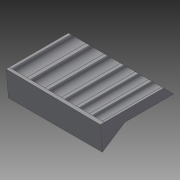
# Autodesk Inventor part: coin_holder
Saved by Autodesk Inventor 2015 (Build 190159000, 159)
## iProperties
Created: 2015-02-10
Part Number: coin_holder
Material: Generic
Document SubType Name: Modeling
Designer: Justin
Density: 1 g/cm^3
Appearance: Default
Author: Justin
Autodesk Inventor part; units mm, degrees
ref_plane "YZ Plane" through (0, 0, 0) normal (1, 0, 0) x (0, 1, 0)
ref_plane "XZ Plane" through (0, 0, 0) normal (0, 1, 0) x (-1, 0, 0)
sketch "Sketch1" plane through (0, 0, 0) normal (0, 0, 1) x (1, 0, 0)
  arc A0 (12.7973, -6.8176) -> (-12.597, -7.1809) centre (0, 0) ccw
  arc A1 (50.4829, -6.2785) -> (26.2017, -6.6259) centre (38.25, 0) ccw
  arc A2 (85.5853, -5.7763) -> (63.5844, -6.091) centre (74.5, 0) ccw
  arc A3 (117.8988, -5.314) -> (98.5072, -5.5914) centre (108.125, 0) ccw
  arc A4 (147.9764, -4.8837) -> (130.6669, -5.1313) centre (139.25, 0) ccw
  arc A5 (177.1345, -4.4665) -> (160.4967, -4.7045) centre (168.75, 0) ccw
  line L0 (-20, 20) -> (188.75, 20)
  line L1 (188.75, 20) -> (188.75, -4.3003)
  line L2 (-20, 20) -> (-20, -7.2868)
  line L3 (-20, -7.2868) -> (188.75, -4.3003)
  dimension "d0" = 29
  dimension "d1" = 27.5
  dimension "d2" = 25
  dimension "d3" = 22.25
  dimension "d4" = 20
  dimension "d5" = 19
  dimension "d6" = 38.25
  dimension "d7" = 36.25
  dimension "d8" = 33.625
  dimension "d9" = 31.125
  dimension "d10" = 29.5
  dimension "d11" = 0
  dimension "d12" = 0
  dimension "d13" = 0
  dimension "d14" = 0
  dimension "d15" = 0
  dimension "d20" = 20
  dimension "d22" = 20
  dimension "d23" = 20
  dimension "d24" = 7
  dimension "d25" = 4.586
  constraints: 12 point on circle, 6 centre point, 6 end point, 1 coincident, 1 horizontal, 1 perpendicular, 1 vertical, 15 other
  measures "d0" diameter of A0
  measures "d1" diameter of A1
  measures "d2" diameter of A2
  measures "d3" diameter of A3
  measures "d4" diameter of A4
  measures "d5" diameter of A5
  measures "d6" distance of A1.centre A0.centre
  measures "d7" distance of A2.centre A1.centre
  measures "d8" distance of A3.centre A2.centre
  measures "d9" distance of A4.centre A3.centre
  measures "d10" distance of A5.centre A4.centre
  measures "d11" vertical distance of point (0, 0) A1.centre
  measures "d12" vertical distance of A1.centre A2.centre
  measures "d13" vertical distance of A2.centre A3.centre
  measures "d14" vertical distance of A3.centre A4.centre
  measures "d15" vertical distance of A4.centre A5.centre
  measures "d20" distance from line of L0 A0.centre
  measures "d22" horizontal distance of A5.centre L0.end
  measures "d23" distance from line of L2 A0.centre
sketch "Sketch4" plane through (0, 0, 0) normal (1, 0, 0) x (0, 1, 0)
  line L0 (0, 0) -> (29.9033, -29.9033)
  line L1 (0, 5.9807) -> (0, -35.884) projected
  point P0 (100, 0)
  dimension "d51" = 45
  dimension "d53" = 0
  dimension "d55" = 29.9033
  dimension "d98" = 100
  constraints: 2 end point
  measures "d51" angle of L0 L1
  measures "d53" vertical distance of L0.start point (100, 0)
  measures "d55" horizontal distance of L0.start L0.end
  measures "d98" distance of L0.start point (100, 0)
ref_plane "Work Plane4" through (0, 100, 0) normal (0, 0.7071068, 0.7071068) x (1, 0, 0)
ref_plane "Work Plane3" through (-10, 0, 0) normal (0, 0.7071068, 0.7071068) x (1, 0, 0)
sketch "Sketch5" plane through (-10, 0, 0) normal (0, 0.7071068, 0.7071068) x (1, 0, 0)
  arc A0 (39.5473, 0.4692) -> (14.153, 0.1059) centre (26.75, 7.2868) ccw
  arc A1 (69.4829, 1.0084) -> (45.2017, 0.661) centre (57.25, 7.2868) ccw
  arc A2 (96.8353, 1.5106) -> (74.8344, 1.1958) centre (85.75, 7.2868) ccw
  arc A3 (121.3988, 1.9729) -> (102.0072, 1.6954) centre (111.625, 7.2868) ccw
  arc A4 (143.7264, 2.4032) -> (126.4169, 2.1555) centre (135, 7.2868) ccw
  arc A5 (165.1345, 2.8203) -> (148.4967, 2.5823) centre (156.75, 7.2868) ccw
  line L0 (10, 27.2868) -> (168.5, 27.2868)
  line L1 (168.5, 27.2868) -> (168.5, 2.9865)
  line L2 (10, 27.2868) -> (10, 0)
  line L3 (10, 0) -> (14.153, 0.1059)
  line L4 (39.5473, 0.4692) -> (45.2017, 0.661)
  line L5 (69.4829, 1.0084) -> (74.8344, 1.1958)
  line L6 (96.8353, 1.5106) -> (102.0072, 1.6954)
  line L7 (165.1345, 2.8203) -> (168.5, 2.9865)
  line L8 (121.3988, 1.9729) -> (126.4169, 2.1555)
  line L9 (143.7264, 2.4032) -> (148.4967, 2.5823)
  dimension "d56" = 29
  dimension "d57" = 27.5
  dimension "d58" = 25
  dimension "d59" = 22.25
  dimension "d60" = 20
  dimension "d61" = 19
  dimension "d62" = 30.5
  dimension "d63" = 28.5
  dimension "d64" = 25.875
  dimension "d65" = 23.375
  dimension "d66" = 21.75
  dimension "d67" = 0
  dimension "d68" = 0
  dimension "d69" = 0
  dimension "d70" = 0
  dimension "d71" = 0
  dimension "d72" = 20
  dimension "d73" = 11.75
  dimension "d74" = 16.75
  constraints: 20 end point, 12 point on circle, 6 centre point, 2 coincident, 1 horizontal, 1 perpendicular, 1 vertical
  measures "d56" diameter of A0
  measures "d57" diameter of A1
  measures "d58" diameter of A2
  measures "d59" diameter of A3
  measures "d60" diameter of A4
  measures "d61" diameter of A5
  measures "d62" distance of A1.centre A0.centre
  measures "d63" distance of A2.centre A1.centre
  measures "d64" distance of A3.centre A2.centre
  measures "d65" distance of A4.centre A3.centre
  measures "d66" distance of A5.centre A4.centre
  measures "d67" vertical distance of point (26.75, 7.287) A1.centre
  measures "d68" vertical distance of A1.centre A2.centre
  measures "d69" vertical distance of A2.centre A3.centre
  measures "d70" vertical distance of A3.centre A4.centre
  measures "d71" vertical distance of A4.centre A5.centre
  measures "d72" distance from line of L0 A0.centre
  measures "d73" horizontal distance of A5.centre L0.end
  measures "d74" distance from line of L2 A0.centre
sketch "Sketch6" plane through (0, 100, 0) normal (0, 0.7071068, 0.7071068) x (1, 0, 0)
  arc A0 (29.5473, 0.4692) -> (4.153, 0.1059) centre (16.75, 7.2868) ccw
  arc A1 (59.4829, 1.0084) -> (35.2017, 0.661) centre (47.25, 7.2868) ccw
  arc A2 (86.8353, 1.5106) -> (64.8344, 1.1958) centre (75.75, 7.2868) ccw
  arc A3 (111.3988, 1.9729) -> (92.0072, 1.6954) centre (101.625, 7.2868) ccw
  arc A4 (133.7264, 2.4032) -> (116.4169, 2.1555) centre (125, 7.2868) ccw
  arc A5 (155.1345, 2.8203) -> (138.4967, 2.5823) centre (146.75, 7.2868) ccw
  line L0 (0, 27.2868) -> (158.5, 27.2868)
  line L1 (158.5, 27.2868) -> (158.5, 2.9865)
  line L2 (0, 27.2868) -> (0, 0)
  line L3 (0, 0) -> (4.153, 0.1059)
  line L4 (29.5473, 0.4692) -> (35.2017, 0.661)
  line L5 (59.4829, 1.0084) -> (64.8344, 1.1958)
  line L6 (86.8353, 1.5106) -> (92.0072, 1.6954)
  line L7 (111.3988, 1.9729) -> (116.4169, 2.1555)
  line L8 (133.7264, 2.4032) -> (138.4967, 2.5823)
  line L9 (155.1345, 2.8203) -> (158.5, 2.9865)
  point P0 (0, -70.7107)
  dimension "d77" = 29
  dimension "d78" = 27.5
  dimension "d79" = 25
  dimension "d80" = 22.25
  dimension "d81" = 20
  dimension "d82" = 19
  dimension "d83" = 30.5
  dimension "d84" = 28.5
  dimension "d85" = 25.875
  dimension "d86" = 23.375
  dimension "d87" = 21.75
  dimension "d88" = 0
  dimension "d89" = 0
  dimension "d90" = 0
  dimension "d91" = 0
  dimension "d92" = 0
  dimension "d93" = 20
  dimension "d94" = 11.75
  dimension "d95" = 16.75
  constraints: 20 end point, 12 point on circle, 6 centre point, 2 coincident, 1 horizontal, 1 perpendicular, 1 vertical
  measures "d77" diameter of A0
  measures "d78" diameter of A1
  measures "d79" diameter of A2
  measures "d80" diameter of A3
  measures "d81" diameter of A4
  measures "d82" diameter of A5
  measures "d83" distance of A1.centre A0.centre
  measures "d84" distance of A2.centre A1.centre
  measures "d85" distance of A3.centre A2.centre
  measures "d86" distance of A4.centre A3.centre
  measures "d87" distance of A5.centre A4.centre
  measures "d88" vertical distance of point (16.75, 7.287) A1.centre
  measures "d89" vertical distance of A1.centre A2.centre
  measures "d90" vertical distance of A2.centre A3.centre
  measures "d91" vertical distance of A3.centre A4.centre
  measures "d92" vertical distance of A4.centre A5.centre
  measures "d93" distance from line of L0 A0.centre
  measures "d94" horizontal distance of A5.centre L0.end
  measures "d95" distance from line of L2 A0.centre
loft "Loft1" add profiles "Sketch6", "Sketch5"
sketch "Sketch7" plane through (0, 0, 0) normal (0, 1, 0) x (-1, 0, 0)
  line L0 (0, 0) -> (0, -19.2947) projected
  line L1 (0, -19.2947) -> (-158.5, -19.2947) projected
  line L2 (-158.5, -19.2947) -> (-158.5, -2.1118) projected
  line L3 (-158.5, -2.1118) -> (-155.1345, -1.9943) projected
  ellipse E0 centre (-146.75, -5.1526) end of major axis (-156.25, -5.1526) minor radius 6.7175 (-155.1345, -1.9943) -> (-138.4967, -1.826) ccw projected
  line L4 (-138.4967, -1.826) -> (-133.7264, -1.6993) projected
  ellipse E1 centre (-125, -5.1526) end of major axis (-135, -5.1526) minor radius 7.0711 (-133.7264, -1.6993) -> (-116.4169, -1.5242) ccw projected
  line L5 (-116.4169, -1.5242) -> (-111.3988, -1.395) projected
  ellipse E2 centre (-101.625, -5.1526) end of major axis (-112.75, -5.1526) minor radius 7.8666 (-111.3988, -1.395) -> (-92.0072, -1.1989) ccw projected
  line L6 (-92.0072, -1.1989) -> (-86.8353, -1.0681) projected
  ellipse E3 centre (-75.75, -5.1526) end of major axis (-88.25, -5.1526) minor radius 8.8388 (-86.8353, -1.0681) -> (-64.8344, -0.8456) ccw projected
  line L7 (-64.8344, -0.8456) -> (-59.4829, -0.713) projected
  ellipse E4 centre (-47.25, -5.1526) end of major axis (-61, -5.1526) minor radius 9.7227 (-59.4829, -0.713) -> (-35.2017, -0.4674) ccw projected
  line L8 (-35.2017, -0.4674) -> (-29.5473, -0.3318) projected
  ellipse E5 centre (-16.75, -5.1526) end of major axis (-31.25, -5.1526) minor radius 10.253 (-29.5473, -0.3318) -> (-4.153, -0.0749) ccw projected
  line L9 (-4.153, -0.0749) -> (0, 0) projected
  line L10 (0, 0) -> (0, -19.2947)
  line L11 (0, -19.2947) -> (-158.5, -19.2947)
  line L12 (-158.5, -19.2947) -> (-158.5, -2.1118)
  line L13 (-158.5, -2.1118) -> (0, 0)
  point P0 (0, 0)
  constraints: 8 end point, 1 collinear, 1 perpendicular, 1 vertical, 6 other
sketch "Sketch10" plane through (0, 19.2947, -19.2947) normal (-1, 0, 0) x (0, 0, 1)
  line L0 (19.2947, 80.7053) -> (0, 100) projected
  line L1 (0, 100) -> (0, 0) projected
  line L2 (19.2947, -19.2947) -> (0, 0) projected
  line L3 (19.2947, 80.7053) -> (19.2947, -19.2947) projected
  line L4 (19.2947, -19.2947) -> (19.2947, -24.2947)
  line L5 (0, 0) -> (0, -22.6066)
  line L6 (0, -22.6066) -> (19.2947, -24.2947)
  line L7 (0, -22.6066) -> (-24.9049, -20.4278)
  line L8 (-24.9049, -20.4278) -> (0, 17.5461)
  line L9 (0, 100) -> (0, 0) projected
  line L10 (0, 17.5461) -> (0, 0)
  point P0 (19.2947, -19.2947)
  dimension "d106" = 5
  dimension "d111" = 85
  dimension "d113" = 25
  dimension "d114" = 40
  constraints: 12 end point, 3 vertical, 1 collinear, 1 point on line
  measures "d106" distance of L2.start L4.end
  measures "d111" angle of L5 L6
  measures "d113" distance of L5.end L7.end
  measures "d114" distance from line of L7 L8.end
sketch "Sketch11" plane through (158.5, 2.1118, -2.1118) normal (1, 0, 0) x (0, 0, -1)
  line L0 (17.1829, 117.1829) -> (0, 100) projected
  line L1 (0, 100) -> (0, 0) projected
  line L2 (17.1829, 17.1829) -> (0, 0) projected
  line L3 (17.1829, 117.1829) -> (17.1829, 17.1829) projected
  line L4 (17.1829, 17.1829) -> (0, 0)
  line L5 (10.1119, 10.1119) -> (-0.5876, -0.5876) projected
  line L6 (17.1829, -5.4237) -> (-2.1118, -7.1118) projected
  line L7 (0, 0) -> (0, -6.927)
  line L8 (17.1829, -5.4237) -> (0, -6.927)
  line L9 (17.1829, -5.4237) -> (17.1829, 17.1829)
  line L10 (0, -6.927) -> (17.1829, -5.4237)
  line L11 (17.1829, -5.4237) -> (42.0878, -3.2448)
  line L12 (42.0878, -3.2448) -> (17.1829, 34.5763)
  line L13 (17.1829, 117.1829) -> (17.1829, 17.1829) projected
  line L14 (17.1829, 17.1829) -> (17.1829, 34.5763)
  point P0 (-2.1118, -2.1118)
  point P1 (17.1829, -7.1118)
  point P2 (-0.4125, -0.4125)
  dimension "d115" = 25
  dimension "d116" = 40
  constraints: 16 end point, 5 collinear, 2 point on line, 2 vertical
  measures "d115" distance of L8.start L11.end
  measures "d116" distance of L6.start L12.end
loft "Loft3" add profiles "Sketch10", "Sketch11" contours L4 L6 L5 L2 | L1 L5 L7 L8 / L12 L11 L9 L3 | L2 L9 L6 L7
body "Solid2"
